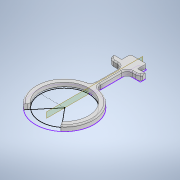
# Autodesk Inventor part: deadbolt enclosure reinforcer from doorknob
Saved by Autodesk Inventor 2022 (Build 260153000, 153)
## iProperties
Created: 2022-04-07
Part Number: deadbolt enclosure reinforcer from doorknob
Material: Generic
Document SubType Name: Modeling
Designer: a-dubs
Density: 1 g/cm^3
Appearance: Default
Author: a-dubs
Autodesk Inventor part; units mm, degrees
ref_plane "YZ Plane" through (0, 0, 0) normal (1, 0, 0) x (0, 1, 0)
ref_plane "XZ Plane" through (0, 0, 0) normal (0, 1, 0) x (-1, 0, 0)
ref_plane "XY Plane" through (0, 0, 0) normal (0, 0, 1) x (1, 0, 0)
sketch "Sketch1" plane through (0, 0, 0) normal (0, 1, 0) x (-1, 0, 0)
  circle A0 centre (0, 0) radius 30.5
  line L0 (0, -30.5) -> (0, -82.5)
  line L1 (0, -82.5) -> (0, -93.5)
  line L2 (0, -93.5) -> (-10.1, -93.5)
  line L3 (-10.1, -93.5) -> (-10.1, -82.5)
  line L4 (-10.1, -82.5) -> (0, -82.5)
  line L5 (-3.0031, -30.5) -> (-3.0031, -30.3518)
  line L6 (-3.0031, -30.5) -> (-3.0031, -82.5)
  line L7 (0, -30.5) -> (-3.0031, -30.5)
  line L8 (-10.1, -82.5) -> (-10.1, -76.1)
  line L9 (-10.1, -76.1) -> (-3.0031, -76.1)
  line L10 (0, -30.5) -> (0, -36.9)
  circle A1 centre (0, 0) radius 36.9
  line L11 (0, 0) -> (23.7189, 28.267)
  line L12 (0, 0) -> (36.9, 0) construction
  line L13 (0, 0) -> (-23.7189, 28.267)
  line L14 (0, 0) -> (36.9, 0) construction
  line L15 (-10.1, -82.5) -> (-19.7, -82.5)
  line L16 (-19.7, -82.5) -> (-19.7, -76.1)
  line L17 (-19.7, -76.1) -> (-10.1, -76.1)
  point P0 (-19.605, 23.3644)
  point P1 (-3.0031, -36.7776)
  point P2 (19.605, 23.3644)
  dimension "d0" = 61
  dimension "d1" = 52
  dimension "d2" = 11
  dimension "d4" = 10.1
  dimension "d8" = 3.0031
  dimension "d9" = 6.4
  dimension "d10" = 6.4
  dimension "d11" = 50
  dimension "d12" = 130
  dimension "d15" = 9.6
  constraints: 36 end point, 5 point on circle, 5 vertical, 4 horizontal, 4 perpendicular, 4 point on line, 2 centre point, 2 coincident, 2 equal length, 1 tangent
  measures "d0" diameter of A0
  measures "d1" distance of L0.start L0.end
  measures "d2" distance of L0.end L1.end
  measures "d4" distance of L1.end L2.end
  measures "d8" distance of L0.start L5.start
  measures "d9" distance of L3.end L8.end
  measures "d10" distance of L0.start L10.end
  measures "d11" angle of L12 L11
  measures "d12" angle of L14 L13
  measures "d15" distance of L3.end L15.end
extrude "Extrusion1" add sketch "Sketch1" along normal blind 6.4 contours L5 L6 A1 L13 A0 | A0 L7 L5 | L0 A1 L6 L7 | L0 L4 L6 A1 | L1 L2 L3 L4 | L6 L4 L8 L9 | L8 L15 L16 L17
fillet "Fillet1" radius 6.4 1 edges at (3.0031, 3.2, -76.1)
chamfer "Chamfer1" distance 3.2 angle 45 1 edges at (19.7, 3.2, -76.1)
fillet "Fillet2" radius 6.4 1 edges at (16.5, 3.2, -76.1)
fillet "Fillet3" radius 6.4 1 edges at (3.0031, 3.2, -36.7776)
ref_plane "Work Plane1" through (0, 3.2, -93.5) normal (-1, 0, 0) x (0, 0, 1)
fillet "Fillet4" radius 1.6 6 edges at (3.0031, 6.4, -55.9833) (4.4103, 6.4, -38.2626) (35.8458, 6.4, -8.7574) (19.0373, 6.4, -78.6373) (4.8776, 6.4, -74.2255) (10.1, 3.2, -93.5)
mirror "Mirror1" about plane through (0, 3.2, -93.5) normal (-1, 0, 0) of "Extrusion1", "Fillet3", "Fillet4", "Fillet2", "Chamfer1", "Fillet1"
chamfer "Chamfer2" distance 1.6 angle 45 5 edges at (0, 0, -93.5) (-9.6314, 0, -93.0314) (-10.1, 0, -87.2) (9.6314, 0, -93.0314) (10.1, 0, -87.2)
chamfer "Chamfer3" distance 1.6 angle 45 1 edges at (0, 0, -30.5)
fillet "Fillet6" radius 3.2 2 edges at (-19.605, 4, 23.3644) (19.605, 4, 23.3644)
body "Solid1"
